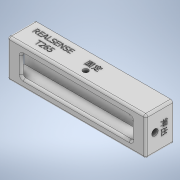
# Autodesk Inventor part: Part1
Saved by Autodesk Inventor 2021.4 (Build 254397000, 397)
## iProperties
Created: 2023-11-13
Part Number: Part1
Material: 一般
Document SubType Name: Modeling
Designer: ryusei
Density: 1 g/cm^3
Appearance: 既定
Author: ryusei
Autodesk Inventor part; units mm, degrees
ref_plane "YZ Plane" through (0, 0, 0) normal (1, 0, 0) x (0, 1, 0)
ref_plane "XZ Plane" through (0, 0, 0) normal (0, 1, 0) x (-1, 0, 0)
ref_plane "XY Plane" through (0, 0, 0) normal (0, 0, 1) x (1, 0, 0)
sketch "スケッチ1" plane through (0, 0, 0) normal (0, 0, 1) x (1, 0, 0)
  line L0 (-64, 17.5) -> (64, 17.5)
  line L1 (64, 17.5) -> (64, -17.5)
  line L2 (64, -17.5) -> (-64, -17.5)
  line L3 (-64, -17.5) -> (-64, 17.5)
  line L4 (-64, 17.5) -> (64, -17.5) construction
  line L5 (64, 17.5) -> (-64, -17.5) construction
  point P0 (0, 0)
  dimension "d0" = 128
  dimension "d1" = 35
  constraints: 12 end point, 2 midpoint, 2 parallel, 1 horizontal, 1 perpendicular
  measures "d0" distance of L1.end L2.end
  measures "d1" distance of L0.end L1.end
extrude "押し出し1" add sketch "スケッチ1" along normal blind 25
sketch "スケッチ3" plane through (-64, -17.5, 0) normal (-1, 0, 0) x (0, 0, 1)
  line L0 (9, 30.5) -> (23, 30.5)
  line L1 (23, 30.5) -> (23, 4.5)
  line L2 (23, 4.5) -> (9, 4.5)
  line L3 (9, 4.5) -> (9, 30.5)
  line L4 (0, 0) -> (25, 0) projected
  line L5 (25, 35) -> (25, 0) projected
  point P0 (0, 17.5)
  dimension "d8" = 14
  dimension "d9" = 26
  dimension "d10" = 4.5
  dimension "d11" = 2
  constraints: 8 end point, 2 parallel, 1 horizontal, 1 perpendicular
  measures "d8" distance of L1.end L2.end
  measures "d9" distance of L0.end L1.end
  measures "d10" distance between parallel lines of L4 L2
  measures "d11" distance between parallel lines of L5 L1
extrude "押し出し2" cut sketch "スケッチ3" against normal blind 118
sketch "スケッチ4" plane through (0, 0, 25) normal (0, 0, 1) x (1, 0, 0)
  line L0 (-51, 9.5) -> (51, 9.5)
  line L1 (51, 9.5) -> (51, -9.5)
  line L2 (51, -9.5) -> (-51, -9.5)
  line L3 (-51, -9.5) -> (-51, 9.5)
  line L4 (-51, 9.5) -> (51, -9.5) construction
  line L5 (51, 9.5) -> (-51, -9.5) construction
  point P0 (0, 0)
  dimension "d14" = 102
  dimension "d15" = 19
  constraints: 12 end point, 2 midpoint, 2 parallel, 1 horizontal, 1 perpendicular
  measures "d14" distance of L0.start L0.end
  measures "d15" distance of L0.end L1.end
extrude "押し出し3" cut sketch "スケッチ4" against normal blind 2
sketch "スケッチ6" plane through (64, -17.5, 0) normal (1, 0, 0) x (0, 0, -1)
  line L0 (0, 0) -> (-25, 0) projected
  line L1 (0, 0) -> (0, 35) projected
  line L2 (-25, 0) -> (-25, 35) projected
  point P0 (0, 17.5)
  point P1 (-16.5, 17.5)
  dimension "d27" = 17.5
  dimension "d46" = 8.5
  measures "d27" distance from line of L0 point (-16.5, 17.5)
  measures "d46" distance from line of L2 point (-16.5, 17.5)
hole "穴2" at (64, 0, 16.5) direction (-1, 0, 0) diameter 6 end through all
sketch "スケッチ7" plane through (-64, 17.5, 0) normal (0, 1, 0) x (1, 0, 0)
  line L0 (128, 0) -> (0, 0) projected
  line L1 (128, 0) -> (128, -25) projected
  line L2 (128, -25) -> (0, -25) projected
  point P0 (64, 0)
  point P1 (64, -16.5)
  dimension "d37" = 64
  dimension "d45" = 8.5
  measures "d37" distance from line of L1 point (64, -16.5)
  measures "d45" distance from line of L2 point (64, -16.5)
hole "穴3" at (0, 17.5, 16.5) direction (0, -1, 0) diameter 4.9 depth 8
sketch "スケッチ8" plane through (-64, -13, 9) normal (0, 0, 1) x (1, 0, 0)
  point P0 (64, 13)
  point P1 (29, 13)
  point P2 (99, 13)
  dimension "d47" = 35
  dimension "d48" = 35
  measures "d47" distance of point (29, 13) point (64, 13)
  measures "d48" distance of point (99, 13) point (64, 13)
hole "穴4" at (-35, 0, 9) at (35, 0, 9) direction (0, 0, -1) diameter 6 depth 15 counterbore diameter 10 counterbore depth 6
fillet "フィレット1" radius 2 12 edges at (-64, 17.5, 12.5) (0, 17.5, 25) (0, -17.5, 25) (-64, -17.5, 12.5) (64, 17.5, 12.5) (-64, 0, 25) (64, 0, 25) (64, -17.5, 12.5) (-51, 9.5, 24) (-51, -9.5, 24) (51, -9.5, 24) (51, 9.5, 24)
fillet "フィレット2" radius 2 8 edges at (50.4142, 8.9142, 25) (51, 0, 25) (50.4142, -8.9142, 25) (0, -9.5, 25) (-50.4142, -8.9142, 25) (-51, 0, 25) (-50.4142, 8.9142, 25) (0, 9.5, 25)
sketch "スケッチ9" plane through (-62, 17.5, 0) normal (0, 1, 0) x (1, 0, 0)
  line L0 (59.5, -8.4717) -> (64.5, -8.4717) construction
  line L1 (64.5, -8.4717) -> (64.5, -10) construction
  line L2 (64.5, -10) -> (59.5, -10) construction
  line L3 (59.5, -10) -> (59.5, -8.4717) construction
  line L4 (0, -25) -> (124, -25) projected
  line L5 (-2, 0) -> (-2, -23) projected
  line L6 (56.3598, -11.9081) -> (56.3598, -12.2565)
  line L7 (56.3598, -12.2565) -> (55.8209, -12.2565)
  line L8 (55.8209, -12.2565) -> (55.8209, -6.4016)
  line L9 (55.8209, -6.4016) -> (61.3274, -6.4016)
  line L10 (61.3274, -6.4016) -> (61.3274, -12.1512)
  line L11 (61.3274, -12.1512) -> (60.7925, -12.1512)
  line L12 (60.7925, -12.1512) -> (60.7925, -11.9081)
  line L13 (60.7925, -11.9081) -> (56.3598, -11.9081)
  line L14 (56.3598, -11.3975) -> (60.7925, -11.3975)
  line L15 (60.7925, -11.3975) -> (60.7925, -6.9121)
  line L16 (60.7925, -6.9121) -> (56.3598, -6.9121)
  line L17 (56.3598, -6.9121) -> (56.3598, -11.3975)
  spline S0 degree 2 poles (58.8314, -7.1552) (59.0462, -7.1795) (58.8558, -7.3132) knots 0 0 0 1 1 1
  line L18 (58.8558, -7.3132) -> (58.8558, -7.7468)
  line L19 (58.8558, -7.7468) -> (60.4684, -7.7468)
  line L20 (60.4684, -7.7468) -> (60.4684, -8.2533)
  line L21 (60.4684, -8.2533) -> (58.8558, -8.2533)
  line L22 (58.8558, -8.2533) -> (58.8558, -8.9786)
  line L23 (58.8558, -8.9786) -> (59.9579, -8.9786)
  line L24 (59.9579, -8.9786) -> (59.9579, -10.9964)
  line L25 (59.9579, -10.9964) -> (59.423, -10.9964)
  line L26 (59.423, -10.9964) -> (59.423, -10.7249)
  line L27 (59.423, -10.7249) -> (57.7577, -10.7249)
  line L28 (57.7577, -10.7249) -> (57.7577, -11.0774)
  line L29 (57.7577, -11.0774) -> (57.2188, -11.0774)
  line L30 (57.2188, -11.0774) -> (57.2188, -8.9786)
  line L31 (57.2188, -8.9786) -> (58.3209, -8.9786)
  line L32 (58.3209, -8.9786) -> (58.3209, -8.2533)
  line L33 (58.3209, -8.2533) -> (56.6556, -8.2533)
  line L34 (56.6556, -8.2533) -> (56.6556, -7.7468)
  line L35 (56.6556, -7.7468) -> (58.3209, -7.7468)
  line L36 (58.3209, -7.7468) -> (58.3209, -7.1552)
  line L37 (58.3209, -7.1552) -> (58.8314, -7.1552)
  line L38 (57.7577, -10.2954) -> (59.423, -10.2954)
  line L39 (59.423, -10.2954) -> (59.423, -9.4121)
  line L40 (59.423, -9.4121) -> (57.7577, -9.4121)
  line L41 (57.7577, -9.4121) -> (57.7577, -10.2954)
  spline S1 degree 2 poles (62.4579, -11.827) (63.7747, -11.0207) (63.7464, -9.25) knots 0 0 0 1 1 1
  line L42 (63.7464, -9.25) -> (64.3622, -9.3554)
  spline S2 degree 2 poles (64.3622, -9.3554) (64.4433, -9.4364) (64.3096, -9.5175) knots 0 0 0 1 1 1
  line L43 (64.3096, -9.5175) -> (64.1759, -10.4858)
  spline S3 degree 2 poles (64.1759, -10.4858) (64.577, -10.968) (65.2212, -11.3165) knots 0 0 0 1 1 1
  line L44 (65.2212, -11.3165) -> (65.2212, -8.7111)
  line L45 (65.2212, -8.7111) -> (63.3979, -8.7111)
  line L46 (63.3979, -8.7111) -> (63.3979, -8.2006)
  line L47 (63.3979, -8.2006) -> (67.4538, -8.2006)
  line L48 (67.4538, -8.2006) -> (67.4538, -8.7111)
  line L49 (67.4538, -8.7111) -> (65.7601, -8.7111)
  line L50 (65.7601, -8.7111) -> (65.7601, -9.7038)
  line L51 (65.7601, -9.7038) -> (67.6402, -9.7038)
  line L52 (67.6402, -9.7038) -> (67.6402, -10.2144)
  line L53 (67.6402, -10.2144) -> (65.7601, -10.2144)
  line L54 (65.7601, -10.2144) -> (65.7601, -11.5069)
  spline S4 degree 2 poles (65.7601, -11.5069) (66.1613, -11.6123) (66.5665, -11.6123) knots 0 0 0 1 1 1
  line L55 (66.5665, -11.6123) -> (68.3371, -11.6123)
  line L56 (68.3371, -11.6123) -> (68.2318, -12.1228)
  line L57 (68.2318, -12.1228) -> (66.5665, -12.1228)
  spline S5 degree 2 poles (66.5665, -12.1228) (65.0065, -12.1228) (64.0138, -10.9964) knots 0 0 0 1 1 1
  spline S6 degree 2 poles (64.0138, -10.9964) (63.6126, -11.8797) (62.8874, -12.3376) knots 0 0 0 1 1 1
  line L58 (62.8874, -12.3376) -> (62.4579, -11.827)
  line L59 (65.7318, -6.9121) -> (68.2034, -6.9121)
  line L60 (68.2034, -6.9121) -> (68.2034, -8.3343)
  line L61 (68.2034, -8.3343) -> (67.6686, -8.3343)
  line L62 (67.6686, -8.3343) -> (67.6686, -7.4226)
  line L63 (67.6686, -7.4226) -> (63.2075, -7.4226)
  line L64 (63.2075, -7.4226) -> (63.2075, -8.391)
  line L65 (63.2075, -8.391) -> (62.6726, -8.391)
  line L66 (62.6726, -8.391) -> (62.6726, -6.9121)
  line L67 (62.6726, -6.9121) -> (65.1159, -6.9121)
  line L68 (65.1159, -6.9121) -> (65.1159, -6.1341)
  line L69 (65.1159, -6.1341) -> (65.7075, -6.1341)
  spline S7 degree 2 poles (65.7075, -6.1341) (65.9749, -6.1868) (65.7318, -6.3489) knots 0 0 0 1 1 1
  line L70 (65.7318, -6.3489) -> (65.7318, -6.9121)
  point P0 (62, 0)
  dimension "d58" = 5
  dimension "d59" = 15
  dimension "d60" = 61.5
  constraints: 2 other
  measures "d58" distance of L0.start L0.end
  measures "d59" distance between parallel lines of L4 L2
  measures "d60" distance between parallel lines of L3 L5
extrude "押し出し4" cut sketch "スケッチ9" against normal blind 1
sketch "スケッチ10" plane through (64, -15.5, 0) normal (1, 0, 0) x (0, 0, -1)
  line L0 (-9.1711, 16.083) -> (-9.1711, 16.6219)
  line L1 (-9.1711, 16.6219) -> (-8.8227, 16.6219)
  line L2 (-8.8227, 16.6219) -> (-8.8227, 17.5336)
  line L3 (-8.8227, 17.5336) -> (-10.8932, 17.5336)
  line L4 (-10.8932, 17.5336) -> (-10.8932, 18.0725)
  line L5 (-10.8932, 18.0725) -> (-8.8227, 18.0725)
  line L6 (-8.8227, 18.0725) -> (-8.8227, 18.9598)
  line L7 (-8.8227, 18.9598) -> (-9.3332, 18.9598)
  line L8 (-9.3332, 18.9598) -> (-9.3332, 19.4947)
  line L9 (-9.3332, 19.4947) -> (-5.1436, 19.4947)
  line L10 (-5.1436, 19.4947) -> (-5.1436, 16.083)
  line L11 (-5.1436, 16.083) -> (-9.1711, 16.083)
  spline S0 degree 2 poles (-8.6079, 20.9452) (-8.6889, 21.241) (-8.8227, 21.5895) knots 0 0 0 1 1 1
  spline S1 degree 2 poles (-8.8227, 21.5895) (-9.0658, 21.7273) (-8.9037, 21.7799) knots 0 0 0 1 1 1
  line L12 (-8.9037, 21.7799) -> (-8.3121, 21.942)
  spline S2 degree 2 poles (-8.3121, 21.942) (-8.2311, 21.5895) (-8.0447, 20.9452) knots 0 0 0 1 1 1
  line L13 (-8.0447, 20.9452) -> (-6.4847, 20.9452)
  line L14 (-6.4847, 20.9452) -> (-6.4847, 21.8853)
  line L15 (-6.4847, 21.8853) -> (-5.9742, 21.8853)
  line L16 (-5.9742, 21.8853) -> (-5.9742, 20.9452)
  line L17 (-5.9742, 20.9452) -> (-4.7667, 20.9452)
  line L18 (-4.7667, 20.9452) -> (-4.7667, 20.4347)
  spline S3 degree 2 poles (-4.7667, 20.4347) (-4.7667, 20.2483) (-4.9288, 20.4104) knots 0 0 0 1 1 1
  line L19 (-4.9288, 20.4104) -> (-5.9742, 20.4104)
  line L20 (-5.9742, 20.4104) -> (-5.9742, 19.7094)
  line L21 (-5.9742, 19.7094) -> (-6.4847, 19.7094)
  line L22 (-6.4847, 19.7094) -> (-6.4847, 20.4104)
  line L23 (-6.4847, 20.4104) -> (-7.8826, 20.4104)
  spline S4 degree 2 poles (-7.8826, 20.4104) (-7.7773, 20.0619) (-7.6679, 19.7662) knots 0 0 0 1 1 1
  line L24 (-7.6679, 19.7662) -> (-8.1501, 19.6568)
  spline S5 degree 2 poles (-8.1501, 19.6568) (-8.2595, 19.9809) (-8.4215, 20.4104) knots 0 0 0 1 1 1
  line L25 (-8.4215, 20.4104) -> (-10.488, 20.4104)
  spline S6 degree 2 poles (-10.488, 20.4104) (-10.9175, 20.4104) (-10.9175, 20.8399) knots 0 0 0 1 1 1
  line L26 (-10.9175, 20.8399) -> (-10.9175, 21.3504)
  line L27 (-10.9175, 21.3504) -> (-10.4069, 21.4558)
  line L28 (-10.4069, 21.4558) -> (-10.4069, 21.0546)
  spline S7 degree 2 poles (-10.4069, 21.0546) (-10.4069, 20.9452) (-10.3016, 20.9452) knots 0 0 0 1 1 1
  line L29 (-10.3016, 20.9452) -> (-8.6079, 20.9452)
  line L30 (-6.7562, 16.6219) -> (-5.6541, 16.6219)
  line L31 (-5.6541, 16.6219) -> (-5.6541, 17.5336)
  line L32 (-5.6541, 17.5336) -> (-6.7562, 17.5336)
  line L33 (-6.7562, 17.5336) -> (-6.7562, 16.6219)
  line L34 (-6.7562, 18.9598) -> (-6.7562, 18.0725)
  line L35 (-6.7562, 18.0725) -> (-5.6541, 18.0725)
  line L36 (-5.6541, 18.0725) -> (-5.6541, 18.9598)
  line L37 (-5.6541, 18.9598) -> (-6.7562, 18.9598)
  line L38 (-8.3121, 16.6219) -> (-7.2667, 16.6219)
  line L39 (-7.2667, 16.6219) -> (-7.2667, 17.5336)
  line L40 (-7.2667, 17.5336) -> (-8.3121, 17.5336)
  line L41 (-8.3121, 17.5336) -> (-8.3121, 16.6219)
  line L42 (-8.3121, 18.9598) -> (-8.3121, 18.0725)
  line L43 (-8.3121, 18.0725) -> (-7.2667, 18.0725)
  line L44 (-7.2667, 18.0725) -> (-7.2667, 18.9598)
  line L45 (-7.2667, 18.9598) -> (-8.3121, 18.9598)
  spline S8 degree 2 poles (-5.492, 13.9355) (-5.5204, 13.7208) (-5.6541, 13.9112) knots 0 0 0 1 1 1
  line L46 (-5.6541, 13.9112) -> (-7.1047, 13.9112)
  line L47 (-7.1047, 13.9112) -> (-7.1047, 12.3229)
  line L48 (-7.1047, 12.3229) -> (-4.9572, 12.3229)
  line L49 (-4.9572, 12.3229) -> (-4.9572, 11.8123)
  spline S9 degree 2 poles (-4.9572, 11.8123) (-4.9815, 11.5976) (-5.1152, 11.788) knots 0 0 0 1 1 1
  line L50 (-5.1152, 11.788) -> (-7.1047, 11.788)
  line L51 (-7.1047, 11.788) -> (-7.1047, 10.2281)
  line L52 (-7.1047, 10.2281) -> (-5.5204, 10.2281)
  line L53 (-5.5204, 10.2281) -> (-5.5204, 9.7175)
  spline S10 degree 2 poles (-5.5204, 9.7175) (-5.5447, 9.5028) (-5.6825, 9.6932) knots 0 0 0 1 1 1
  line L54 (-5.6825, 9.6932) -> (-7.8583, 9.6932)
  line L55 (-7.8583, 9.6932) -> (-7.8583, 10.2281)
  line L56 (-7.8583, 10.2281) -> (-7.6152, 10.2281)
  line L57 (-7.6152, 10.2281) -> (-7.6152, 11.788)
  line L58 (-7.6152, 11.788) -> (-9.9248, 11.788)
  line L59 (-9.9248, 11.788) -> (-9.9248, 10.0133)
  line L60 (-9.9248, 10.0133) -> (-8.2878, 10.0133)
  line L61 (-8.2878, 10.0133) -> (-8.2878, 9.5028)
  spline S11 degree 2 poles (-8.2878, 9.5028) (-8.3121, 9.288) (-8.4458, 9.4785) knots 0 0 0 1 1 1
  line L62 (-8.4458, 9.4785) -> (-10.7311, 9.4785)
  line L63 (-10.7311, 9.4785) -> (-10.7311, 10.0133)
  line L64 (-10.7311, 10.0133) -> (-10.4353, 10.0133)
  line L65 (-10.4353, 10.0133) -> (-10.4353, 14.1786)
  line L66 (-10.4353, 14.1786) -> (-10.8121, 14.1786)
  line L67 (-10.8121, 14.1786) -> (-10.8121, 14.7135)
  line L68 (-10.8121, 14.7135) -> (-8.2595, 14.7135)
  line L69 (-8.2595, 14.7135) -> (-8.2595, 14.2029)
  spline S12 degree 2 poles (-8.2595, 14.2029) (-8.2878, 13.9882) (-8.4215, 14.1786) knots 0 0 0 1 1 1
  line L70 (-8.4215, 14.1786) -> (-9.9248, 14.1786)
  line L71 (-9.9248, 14.1786) -> (-9.9248, 12.3229)
  line L72 (-9.9248, 12.3229) -> (-7.6152, 12.3229)
  line L73 (-7.6152, 12.3229) -> (-7.6152, 13.9112)
  line L74 (-7.6152, 13.9112) -> (-7.911, 13.9112)
  line L75 (-7.911, 13.9112) -> (-7.911, 14.4461)
  line L76 (-7.911, 14.4461) -> (-5.492, 14.4461)
  line L77 (-5.492, 14.4461) -> (-5.492, 13.9355)
  point P0 (0, 15.5)
  point P1 (-7.8421, 15.4671)
  constraints: 1 other
extrude "押し出し5" cut sketch "スケッチ10" against normal blind 1
sketch "スケッチ11" plane through (-62, 17.5, 0) normal (0, 1, 0) x (1, 0, 0)
  line L0 (-8.9503, -5.0587) -> (55.772, -5.0587) construction
  line L1 (55.772, -5.0587) -> (55.772, -11.4158) construction
  line L2 (55.772, -11.4158) -> (-8.9503, -11.4158) construction
  line L3 (-8.9503, -11.4158) -> (-8.9503, -5.0587) construction
  line L4 (9.9708, -10.1479) -> (9.1077, -10.1479)
  line L5 (9.1077, -10.1479) -> (7.5275, -8.1584)
  line L6 (7.5275, -8.1584) -> (6.7658, -8.1584)
  line L7 (6.7658, -8.1584) -> (6.7658, -10.1479)
  line L8 (6.7658, -10.1479) -> (6.1013, -10.1479)
  line L9 (6.1013, -10.1479) -> (6.1013, -5.1479)
  line L10 (6.1013, -5.1479) -> (7.3897, -5.1479)
  spline S0 degree 2 poles (7.3897, -5.1479) (7.8192, -5.1479) (8.3987, -5.2411) (8.662, -5.4113) knots 0 0 0 1 2 2 2
  spline S1 degree 2 poles (8.662, -5.4113) (8.9254, -5.5814) (9.2293, -6.1122) (9.2293, -6.5053) knots 0 0 0 1 2 2 2
  spline S2 degree 2 poles (9.2293, -6.5053) (9.2293, -7.0523) (8.6701, -7.7937) (8.192, -7.972) knots 0 0 0 1 2 2 2
  line L11 (8.192, -7.972) -> (9.9708, -10.1479)
  spline S3 degree 2 poles (8.5364, -6.5579) (8.5364, -6.3391) (8.3825, -6.0028) (8.2204, -5.8934) knots 0 0 0 1 2 2 2
  spline S4 degree 2 poles (8.2204, -5.8934) (8.0786, -5.8002) (7.7017, -5.7232) (7.4262, -5.7232) knots 0 0 0 1 2 2 2
  line L12 (7.4262, -5.7232) -> (6.7658, -5.7232)
  line L13 (6.7658, -5.7232) -> (6.7658, -7.6033)
  line L14 (6.7658, -7.6033) -> (7.3492, -7.6033)
  spline S5 degree 2 poles (7.3492, -7.6033) (7.6369, -7.6033) (8.0948, -7.502) (8.2528, -7.344) knots 0 0 0 1 2 2 2
  spline S6 degree 2 poles (8.2528, -7.344) (8.3987, -7.2062) (8.5364, -6.8172) (8.5364, -6.5579) knots 0 0 0 1 2 2 2
  line L15 (10.3679, -10.1479) -> (10.3679, -5.1479)
  line L16 (10.3679, -5.1479) -> (13.4959, -5.1479)
  line L17 (13.4959, -5.1479) -> (13.4959, -5.7395)
  line L18 (13.4959, -5.7395) -> (11.0324, -5.7395)
  line L19 (11.0324, -5.7395) -> (11.0324, -7.109)
  line L20 (11.0324, -7.109) -> (13.3298, -7.109)
  line L21 (13.3298, -7.109) -> (13.3298, -7.7006)
  line L22 (13.3298, -7.7006) -> (11.0324, -7.7006)
  line L23 (11.0324, -7.7006) -> (11.0324, -9.5563)
  line L24 (11.0324, -9.5563) -> (13.4959, -9.5563)
  line L25 (13.4959, -9.5563) -> (13.4959, -10.1479)
  line L26 (13.4959, -10.1479) -> (10.3679, -10.1479)
  line L27 (13.6863, -10.1479) -> (15.3719, -5.1479)
  line L28 (15.3719, -5.1479) -> (16.1904, -5.1479)
  line L29 (16.1904, -5.1479) -> (17.876, -10.1479)
  line L30 (17.876, -10.1479) -> (17.175, -10.1479)
  line L31 (17.175, -10.1479) -> (16.7212, -8.75)
  line L32 (16.7212, -8.75) -> (14.8128, -8.75)
  line L33 (14.8128, -8.75) -> (14.359, -10.1479)
  line L34 (14.359, -10.1479) -> (13.6863, -10.1479)
  line L35 (16.5389, -8.1827) -> (15.7649, -5.8286)
  line L36 (15.7649, -5.8286) -> (14.9951, -8.1827)
  line L37 (14.9951, -8.1827) -> (16.5389, -8.1827)
  line L38 (21.2471, -10.1479) -> (18.35, -10.1479)
  line L39 (18.35, -10.1479) -> (18.35, -5.1479)
  line L40 (18.35, -5.1479) -> (19.0145, -5.1479)
  line L41 (19.0145, -5.1479) -> (19.0145, -9.5563)
  line L42 (19.0145, -9.5563) -> (21.2471, -9.5563)
  line L43 (21.2471, -9.5563) -> (21.2471, -10.1479)
  spline S7 degree 2 poles (23.1637, -10.237) (22.6207, -10.237) (21.859, -10.0101) (21.5226, -9.848) knots 0 0 0 1 2 2 2
  line L44 (21.5226, -9.848) -> (21.5226, -9.0134)
  line L45 (21.5226, -9.0134) -> (21.5713, -9.0134)
  spline S8 degree 2 poles (21.5713, -9.0134) (21.8995, -9.3213) (22.7301, -9.6617) (23.115, -9.6617) knots 0 0 0 1 2 2 2
  spline S9 degree 2 poles (23.115, -9.6617) (23.6661, -9.6617) (24.2293, -9.2038) (24.2293, -8.827) knots 0 0 0 1 2 2 2
  spline S10 degree 2 poles (24.2293, -8.827) (24.2293, -8.5271) (23.9335, -8.1544) (23.6134, -8.0612) knots 0 0 0 1 2 2 2
  spline S11 degree 2 poles (23.6134, -8.0612) (23.3825, -7.9963) (22.9975, -7.9072) (22.7098, -7.8343) knots 0 0 0 1 2 2 2
  spline S12 degree 2 poles (22.7098, -7.8343) (22.4505, -7.7654) (22.0413, -7.5587) (21.8833, -7.3926) knots 0 0 0 1 2 2 2
  spline S13 degree 2 poles (21.8833, -7.3926) (21.7293, -7.2265) (21.5591, -6.7808) (21.5591, -6.489) knots 0 0 0 1 2 2 2
  spline S14 degree 2 poles (21.5591, -6.489) (21.5591, -5.8813) (22.5073, -5.0587) (23.2406, -5.0587) knots 0 0 0 1 2 2 2
  spline S15 degree 2 poles (23.2406, -5.0587) (23.662, -5.0587) (24.4076, -5.2249) (24.7277, -5.3829) knots 0 0 0 1 2 2 2
  line L46 (24.7277, -5.3829) -> (24.7277, -6.1771)
  line L47 (24.7277, -6.1771) -> (24.679, -6.1771)
  spline S16 degree 2 poles (24.679, -6.1771) (24.44, -5.9583) (23.6944, -5.6341) (23.2852, -5.6341) knots 0 0 0 1 2 2 2
  spline S17 degree 2 poles (23.2852, -5.6341) (22.8233, -5.6341) (22.252, -6.0677) (22.252, -6.4202) knots 0 0 0 1 2 2 2
  spline S18 degree 2 poles (22.252, -6.4202) (22.252, -6.7362) (22.5883, -7.113) (22.9043, -7.1981) knots 0 0 0 1 2 2 2
  spline S19 degree 2 poles (22.9043, -7.1981) (23.115, -7.2549) (23.7269, -7.4007) (23.9295, -7.4615) knots 0 0 0 1 2 2 2
  spline S20 degree 2 poles (23.9295, -7.4615) (24.444, -7.6195) (24.9222, -8.2557) (24.9222, -8.7216) knots 0 0 0 1 2 2 2
  spline S21 degree 2 poles (24.9222, -8.7216) (24.9222, -9.0174) (24.6831, -9.5847) (24.4684, -9.7832) knots 0 0 0 1 2 2 2
  spline S22 degree 2 poles (24.4684, -9.7832) (24.2293, -10.002) (23.6215, -10.237) (23.1637, -10.237) knots 0 0 0 1 2 2 2
  line L48 (25.5988, -10.1479) -> (25.5988, -5.1479)
  line L49 (25.5988, -5.1479) -> (28.7269, -5.1479)
  line L50 (28.7269, -5.1479) -> (28.7269, -5.7395)
  line L51 (28.7269, -5.7395) -> (26.2633, -5.7395)
  line L52 (26.2633, -5.7395) -> (26.2633, -7.109)
  line L53 (26.2633, -7.109) -> (28.5607, -7.109)
  line L54 (28.5607, -7.109) -> (28.5607, -7.7006)
  line L55 (28.5607, -7.7006) -> (26.2633, -7.7006)
  line L56 (26.2633, -7.7006) -> (26.2633, -9.5563)
  line L57 (26.2633, -9.5563) -> (28.7269, -9.5563)
  line L58 (28.7269, -9.5563) -> (28.7269, -10.1479)
  line L59 (28.7269, -10.1479) -> (25.5988, -10.1479)
  line L60 (33.034, -10.1479) -> (32.2884, -10.1479)
  line L61 (32.2884, -10.1479) -> (30.0761, -5.8367)
  line L62 (30.0761, -5.8367) -> (30.0761, -10.1479)
  line L63 (30.0761, -10.1479) -> (29.4562, -10.1479)
  line L64 (29.4562, -10.1479) -> (29.4562, -5.1479)
  line L65 (29.4562, -5.1479) -> (30.4003, -5.1479)
  line L66 (30.4003, -5.1479) -> (32.4141, -9.1066)
  line L67 (32.4141, -9.1066) -> (32.4141, -5.1479)
  line L68 (32.4141, -5.1479) -> (33.034, -5.1479)
  line L69 (33.034, -5.1479) -> (33.034, -10.1479)
  spline S23 degree 2 poles (35.4408, -10.237) (34.8979, -10.237) (34.1361, -10.0101) (33.7998, -9.848) knots 0 0 0 1 2 2 2
  line L70 (33.7998, -9.848) -> (33.7998, -9.0134)
  line L71 (33.7998, -9.0134) -> (33.8484, -9.0134)
  spline S24 degree 2 poles (33.8484, -9.0134) (34.1766, -9.3213) (35.0073, -9.6617) (35.3922, -9.6617) knots 0 0 0 1 2 2 2
  spline S25 degree 2 poles (35.3922, -9.6617) (35.9432, -9.6617) (36.5064, -9.2038) (36.5064, -8.827) knots 0 0 0 1 2 2 2
  spline S26 degree 2 poles (36.5064, -8.827) (36.5064, -8.5271) (36.2107, -8.1544) (35.8906, -8.0612) knots 0 0 0 1 2 2 2
  spline S27 degree 2 poles (35.8906, -8.0612) (35.6596, -7.9963) (35.2747, -7.9072) (34.987, -7.8343) knots 0 0 0 1 2 2 2
  spline S28 degree 2 poles (34.987, -7.8343) (34.7277, -7.7654) (34.3184, -7.5587) (34.1604, -7.3926) knots 0 0 0 1 2 2 2
  spline S29 degree 2 poles (34.1604, -7.3926) (34.0064, -7.2265) (33.8363, -6.7808) (33.8363, -6.489) knots 0 0 0 1 2 2 2
  spline S30 degree 2 poles (33.8363, -6.489) (33.8363, -5.8813) (34.7844, -5.0587) (35.5178, -5.0587) knots 0 0 0 1 2 2 2
  spline S31 degree 2 poles (35.5178, -5.0587) (35.9392, -5.0587) (36.6847, -5.2249) (37.0048, -5.3829) knots 0 0 0 1 2 2 2
  line L72 (37.0048, -5.3829) -> (37.0048, -6.1771)
  line L73 (37.0048, -6.1771) -> (36.9562, -6.1771)
  spline S32 degree 2 poles (36.9562, -6.1771) (36.7171, -5.9583) (35.9716, -5.6341) (35.5624, -5.6341) knots 0 0 0 1 2 2 2
  spline S33 degree 2 poles (35.5624, -5.6341) (35.1004, -5.6341) (34.5291, -6.0677) (34.5291, -6.4202) knots 0 0 0 1 2 2 2
  spline S34 degree 2 poles (34.5291, -6.4202) (34.5291, -6.7362) (34.8654, -7.113) (35.1815, -7.1981) knots 0 0 0 1 2 2 2
  spline S35 degree 2 poles (35.1815, -7.1981) (35.3922, -7.2549) (36.004, -7.4007) (36.2066, -7.4615) knots 0 0 0 1 2 2 2
  spline S36 degree 2 poles (36.2066, -7.4615) (36.7212, -7.6195) (37.1993, -8.2557) (37.1993, -8.7216) knots 0 0 0 1 2 2 2
  spline S37 degree 2 poles (37.1993, -8.7216) (37.1993, -9.0174) (36.9602, -9.5847) (36.7455, -9.7832) knots 0 0 0 1 2 2 2
  spline S38 degree 2 poles (36.7455, -9.7832) (36.5064, -10.002) (35.8987, -10.237) (35.4408, -10.237) knots 0 0 0 1 2 2 2
  line L74 (37.876, -10.1479) -> (37.876, -5.1479)
  line L75 (37.876, -5.1479) -> (41.004, -5.1479)
  line L76 (41.004, -5.1479) -> (41.004, -5.7395)
  line L77 (41.004, -5.7395) -> (38.5405, -5.7395)
  line L78 (38.5405, -5.7395) -> (38.5405, -7.109)
  line L79 (38.5405, -7.109) -> (40.8379, -7.109)
  line L80 (40.8379, -7.109) -> (40.8379, -7.7006)
  line L81 (40.8379, -7.7006) -> (38.5405, -7.7006)
  line L82 (38.5405, -7.7006) -> (38.5405, -9.5563)
  line L83 (38.5405, -9.5563) -> (41.004, -9.5563)
  line L84 (41.004, -9.5563) -> (41.004, -10.1479)
  line L85 (41.004, -10.1479) -> (37.876, -10.1479)
  line L86 (17.4485, -18.3803) -> (17.4485, -13.9718)
  line L87 (17.4485, -13.9718) -> (15.771, -13.9718)
  line L88 (15.771, -13.9718) -> (15.771, -13.3803)
  line L89 (15.771, -13.3803) -> (19.7905, -13.3803)
  line L90 (19.7905, -13.3803) -> (19.7905, -13.9718)
  line L91 (19.7905, -13.9718) -> (18.113, -13.9718)
  line L92 (18.113, -13.9718) -> (18.113, -18.3803)
  line L93 (18.113, -18.3803) -> (17.4485, -18.3803)
  line L94 (23.2386, -18.3803) -> (20.1551, -18.3803)
  line L95 (20.1551, -18.3803) -> (20.1551, -17.6712)
  spline S39 degree 2 poles (20.1551, -17.6712) (20.4874, -17.3592) (21.079, -16.7798) (21.3626, -16.4678) knots 0 0 0 1 2 2 2
  spline S40 degree 2 poles (21.3626, -16.4678) (21.9339, -15.8397) (22.3513, -15.0861) (22.3513, -14.685) knots 0 0 0 1 2 2 2
  spline S41 degree 2 poles (22.3513, -14.685) (22.3513, -14.4743) (22.2216, -14.1582) (22.1041, -14.0569) knots 0 0 0 1 2 2 2
  spline S42 degree 2 poles (22.1041, -14.0569) (21.9866, -13.9556) (21.6786, -13.8543) (21.4923, -13.8543) knots 0 0 0 1 2 2 2
  spline S43 degree 2 poles (21.4923, -13.8543) (21.314, -13.8543) (20.9493, -13.9435) (20.7832, -14.0123) knots 0 0 0 1 2 2 2
  spline S44 degree 2 poles (20.7832, -14.0123) (20.6414, -14.0691) (20.378, -14.2311) (20.297, -14.2879) knots 0 0 0 1 2 2 2
  line L96 (20.297, -14.2879) -> (20.2605, -14.2879)
  line L97 (20.2605, -14.2879) -> (20.2605, -13.5747)
  spline S45 degree 2 poles (20.2605, -13.5747) (20.4671, -13.4734) (21.2086, -13.2749) (21.5409, -13.2749) knots 0 0 0 1 2 2 2
  spline S46 degree 2 poles (21.5409, -13.2749) (22.2419, -13.2749) (23.032, -14.0164) (23.032, -14.6485) knots 0 0 0 1 2 2 2
  spline S47 degree 2 poles (23.032, -14.6485) (23.032, -14.9443) (22.8942, -15.4386) (22.7726, -15.6493) knots 0 0 0 1 2 2 2
  spline S48 degree 2 poles (22.7726, -15.6493) (22.6511, -15.8681) (22.2986, -16.2976) (22.1041, -16.5042) knots 0 0 0 1 2 2 2
  spline S49 degree 2 poles (22.1041, -16.5042) (21.788, -16.8486) (21.0141, -17.5861) (20.7832, -17.8008) knots 0 0 0 1 2 2 2
  line L98 (20.7832, -17.8008) -> (23.2386, -17.8008)
  line L99 (23.2386, -17.8008) -> (23.2386, -18.3803)
  spline S50 degree 2 poles (27.0676, -16.7595) (27.0676, -17.1444) (26.8124, -17.7968) (26.5976, -18.0156) knots 0 0 0 1 2 2 2
  spline S51 degree 2 poles (26.5976, -18.0156) (26.3748, -18.2465) (25.8156, -18.4856) (25.4793, -18.4856) knots 0 0 0 1 2 2 2
  spline S52 degree 2 poles (25.4793, -18.4856) (25.143, -18.4856) (24.5879, -18.2587) (24.3772, -18.0318) knots 0 0 0 1 2 2 2
  spline S53 degree 2 poles (24.3772, -18.0318) (24.1179, -17.7603) (23.8261, -16.8486) (23.8261, -16.1841) knots 0 0 0 1 2 2 2
  spline S54 degree 2 poles (23.8261, -16.1841) (23.8261, -15.5318) (24.0936, -14.4824) (24.3731, -14.0934) knots 0 0 0 1 2 2 2
  spline S55 degree 2 poles (24.3731, -14.0934) (24.6446, -13.7125) (25.5036, -13.2871) (26.0668, -13.2871) knots 0 0 0 1 2 2 2
  spline S56 degree 2 poles (26.0668, -13.2871) (26.2329, -13.2871) (26.5247, -13.3195) (26.6341, -13.3559) knots 0 0 0 1 2 2 2
  line L100 (26.6341, -13.3559) -> (26.6341, -14.0002)
  line L101 (26.6341, -14.0002) -> (26.6057, -14.0002)
  spline S57 degree 2 poles (26.6057, -14.0002) (26.5125, -13.9516) (26.1722, -13.8665) (25.9777, -13.8665) knots 0 0 0 1 2 2 2
  spline S58 degree 2 poles (25.9777, -13.8665) (25.3537, -13.8665) (24.5879, -14.7093) (24.5149, -15.5358) knots 0 0 0 1 2 2 2
  spline S59 degree 2 poles (24.5149, -15.5358) (24.754, -15.3697) (25.2564, -15.1874) (25.5563, -15.1874) knots 0 0 0 1 2 2 2
  spline S60 degree 2 poles (25.5563, -15.1874) (25.848, -15.1874) (26.2856, -15.3049) (26.5247, -15.4832) knots 0 0 0 1 2 2 2
  spline S61 degree 2 poles (26.5247, -15.4832) (26.8002, -15.6898) (27.0676, -16.33) (27.0676, -16.7595) knots 0 0 0 1 2 2 2
  spline S62 degree 2 poles (26.3869, -16.7879) (26.3869, -16.4799) (26.2248, -16.0626) (26.0466, -15.9167) knots 0 0 0 1 2 2 2
  spline S63 degree 2 poles (26.0466, -15.9167) (25.9128, -15.8114) (25.5806, -15.7425) (25.4064, -15.7425) knots 0 0 0 1 2 2 2
  spline S64 degree 2 poles (25.4064, -15.7425) (25.1714, -15.7425) (24.7297, -15.8843) (24.5149, -16.018) knots 0 0 0 1 2 2 2
  spline S65 degree 2 poles (24.5149, -16.018) (24.5109, -16.0909) (24.5028, -16.2287) (24.5028, -16.3341) knots 0 0 0 1 2 2 2
  spline S66 degree 2 poles (24.5028, -16.3341) (24.5028, -16.8527) (24.7054, -17.4888) (24.8594, -17.655) knots 0 0 0 1 2 2 2
  spline S67 degree 2 poles (24.8594, -17.655) (25.0012, -17.813) (25.3091, -17.9386) (25.4833, -17.9386) knots 0 0 0 1 2 2 2
  spline S68 degree 2 poles (25.4833, -17.9386) (25.8885, -17.9386) (26.3869, -17.3632) (26.3869, -16.7879) knots 0 0 0 1 2 2 2
  spline S69 degree 2 poles (30.69, -16.7919) (30.69, -17.1525) (30.459, -17.7684) (30.2483, -17.9953) knots 0 0 0 1 2 2 2
  spline S70 degree 2 poles (30.2483, -17.9953) (30.0376, -18.2222) (29.4096, -18.4856) (29.0206, -18.4856) knots 0 0 0 1 2 2 2
  spline S71 degree 2 poles (29.0206, -18.4856) (28.6641, -18.4856) (27.9671, -18.3276) (27.7119, -18.202) knots 0 0 0 1 2 2 2
  line L102 (27.7119, -18.202) -> (27.7119, -17.4929)
  line L103 (27.7119, -17.4929) -> (27.7605, -17.4929)
  spline S72 degree 2 poles (27.7605, -17.4929) (27.8375, -17.5496) (28.1252, -17.6955) (28.2994, -17.7603) knots 0 0 0 1 2 2 2
  spline S73 degree 2 poles (28.2994, -17.7603) (28.4979, -17.8292) (28.8261, -17.9062) (29.0328, -17.9062) knots 0 0 0 1 2 2 2
  spline S74 degree 2 poles (29.0328, -17.9062) (29.2354, -17.9062) (29.6162, -17.7603) (29.754, -17.6023) knots 0 0 0 1 2 2 2
  spline S75 degree 2 poles (29.754, -17.6023) (29.8796, -17.4524) (30.0093, -17.0553) (30.0093, -16.7879) knots 0 0 0 1 2 2 2
  spline S76 degree 2 poles (30.0093, -16.7879) (30.0093, -16.5204) (29.8634, -16.1801) (29.7256, -16.0666) knots 0 0 0 1 2 2 2
  spline S77 degree 2 poles (29.7256, -16.0666) (29.5838, -15.941) (29.1624, -15.8357) (28.9072, -15.8357) knots 0 0 0 1 2 2 2
  spline S78 degree 2 poles (28.9072, -15.8357) (28.6316, -15.8357) (28.0846, -15.9208) (27.9185, -15.9572) knots 0 0 0 1 2 2 2
  line L104 (27.9185, -15.9572) -> (27.9185, -13.3803)
  line L105 (27.9185, -13.3803) -> (30.6616, -13.3803)
  line L106 (30.6616, -13.3803) -> (30.6616, -13.9678)
  line L107 (30.6616, -13.9678) -> (28.5628, -13.9678)
  line L108 (28.5628, -13.9678) -> (28.5628, -15.3008)
  spline S79 degree 2 poles (28.5628, -15.3008) (28.6843, -15.2846) (28.9193, -15.2725) (29.0166, -15.2725) knots 0 0 0 1 2 2 2
  spline S80 degree 2 poles (29.0166, -15.2725) (29.4015, -15.2725) (29.9323, -15.3981) (30.1754, -15.5845) knots 0 0 0 1 2 2 2
  spline S81 degree 2 poles (30.1754, -15.5845) (30.4226, -15.7708) (30.69, -16.3381) (30.69, -16.7919) knots 0 0 0 1 2 2 2
  point P0 (62, 0)
  constraints: 2 other
extrude "押し出し6" cut sketch "スケッチ11" against normal blind 1
